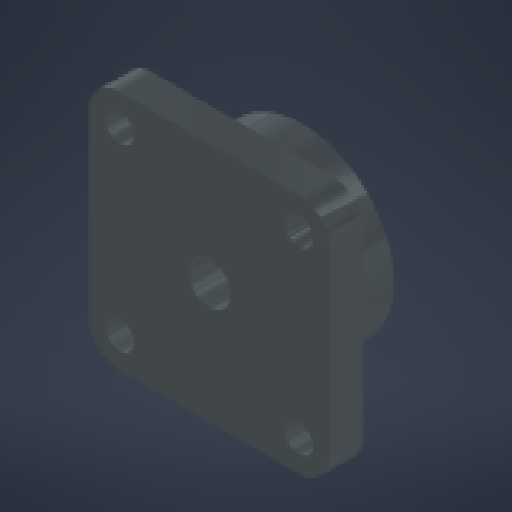
# Autodesk Inventor part: bearing_unit_15mm
Saved by Autodesk Inventor 2026 (Build 300175000, 175)
## iProperties
Created: 2026-05-04
Part Number: bearing_unit_15mm
Material: Чугун, серый
Document SubType Name: Modeling
Designer: user
Density: 7.15 g/cm^3
Appearance: Чугун серый
Mass: 824.689 g
Surface Area: 185.073 cm^2
Volume: 115.341 cm^3
Author: user
Autodesk Inventor part; units mm, degrees
ref_plane "YZ Plane" through (0, 0, 0) normal (1, 0, 0) x (0, 1, 0)
ref_plane "XZ Plane" through (0, 0, 0) normal (0, 1, 0) x (-1, 0, 0)
ref_plane "XY Plane" through (0, 0, 0) normal (0, 0, 1) x (1, 0, 0)
sketch "Эскиз1" plane through (0, 0, 0) normal (0, 0, 1) x (1, 0, 0)
  circle A0 centre (0, 0) radius 7.5
  line L0 (46.4621, 0) -> (-49.3756, 0)
  circle A1 centre (32, -32) radius 5
  line L1 (0, 64.1704) -> (0, -88.8862)
  circle A2 centre (32, 32) radius 5
  circle A3 centre (-32, -32) radius 5
  circle A4 centre (-32, 32) radius 5
  arc A5 (-43, -32) -> (-32, -43) centre (-32, -32) ccw
  arc A6 (-32, 43) -> (-43, 32) centre (-32, 32) ccw
  arc A7 (32, -43) -> (43, -32) centre (32, -32) ccw
  arc A8 (43, 32) -> (32, 43) centre (32, 32) ccw
  line L2 (43, -32) -> (43, 32)
  line L3 (32, 43) -> (-32, 43)
  line L4 (-43, 32) -> (-43, -32)
  line L5 (-32, -43) -> (32, -43)
  dimension "d0" = 15
  dimension "d11" = 10
  dimension "d12" = 64
  dimension "d13" = 64
  dimension "d14" = 22
  constraints: 12 end point, 9 centre point, 8 point on circle, 8 tangent, 4 coincident, 4 symmetric about line, 2 equal radius, 2 point on line, 1 horizontal, 1 vertical, 4 other
  measures "d0" diameter of A0
  measures "d11" diameter of A1
  measures "d12" distance of A2.centre A1.centre
  measures "d13" distance of A3.centre A1.centre
  measures "d14" diameter of A5
extrude "Выдавливание1" add sketch "Эскиз1" along normal blind 12 contours L0 L2 A7 L5 L1 A0 | A0 L1 L3 A8 L2 L0 | A0 L0 L4 A6 L3 L1 | L1 L5 A5 L4 L0 A0
sketch "Эскиз2" plane through (0, 0, 0) normal (0, 0, -1) x (-1, 0, 0)
  circle A0 centre (0, 0) radius 7.5 projected
  line L0 (10.171, 50.3667) -> (28.7441, 15.1667) projected
  circle A1 centre (0, 0) radius 32.5
  constraints: 1 coincident, 3 other
extrude "Выдавливание2" add sketch "Эскиз2" along normal blind 21.3
